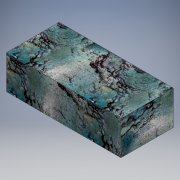
# Autodesk Inventor part: 1550
Saved by Autodesk Inventor 2020 (Build 240168000, 168)
## iProperties
Created: 2024-12-18
Part Number: 1550
Material: Типовые
Document SubType Name: Modeling
Designer: Ivan
Mass: 103000 g
Surface Area: 97.84 cm^2
Volume: 55.352 cm^3
Density: 1860.82 g/cm^3
Appearance: Камень — синий
Author: Ivan
Autodesk Inventor part; units mm, degrees
ref_plane "YZ Plane" through (0, 0, 0) normal (1, 0, 0) x (0, 1, 0)
ref_plane "XZ Plane" through (0, 0, 0) normal (0, 1, 0) x (-1, 0, 0)
ref_plane "XY Plane" through (0, 0, 0) normal (0, 0, 1) x (1, 0, 0)
sketch "Эскиз1" plane through (0, 0, 0) normal (1, 0, 0) x (0, 1, 0)
  line L0 (11, 17) -> (-11, 17)
  line L1 (-11, 17) -> (-11, -17)
  line L2 (-11, -17) -> (11, -17)
  line L3 (11, -17) -> (11, 17)
  line L4 (11, 17) -> (-11, -17) construction
  point P0 (0, 0)
  point P1 (0, 0)
  point P2 (11, 5.6667)
  point P3 (11, -5.6667)
  dimension "d0" = 22
  dimension "d1" = 34
  dimension "d4" = 11.3333
  dimension "d5" = 11.3333
  constraints: 10 end point, 2 parallel, 2 point on line, 1 coincident, 1 horizontal, 1 midpoint, 1 perpendicular
  measures "d0" distance of L2.end L1.end
  measures "d1" distance of L1.end L0.end
  measures "d4" distance from line of point (11, 5.667) L0
  measures "d5" distance from line of point (11, -5.667) L2
extrude "Выдавливание1" add sketch "Эскиз1" against normal blind 74
equation "\"d4\" = 0.333333 * d1"
equation "\"d5\" = d4"
